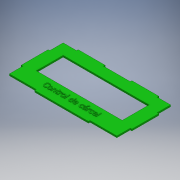
# Autodesk Inventor part: Control Frontal
Saved by Autodesk Inventor 2018 (Build 220112000, 112)
## iProperties
Created: 2020-03-09
Part Number: Control Frontal
Material: Genérico
Document SubType Name: Modeling
Designer: joser
Density: 1 g/cm^3
Appearance: Verde oscuro
Author: joser
Autodesk Inventor part; units mm, degrees
ref_plane "YZ Plane" through (0, 0, 0) normal (1, 0, 0) x (0, 1, 0)
ref_plane "XZ Plane" through (0, 0, 0) normal (0, 1, 0) x (-1, 0, 0)
ref_plane "XY Plane" through (0, 0, 0) normal (0, 0, 1) x (1, 0, 0)
sketch "Boceto1" plane through (0, 0, 0) normal (0, 0, 1) x (1, 0, 0)
  line L0 (-150, -3) -> (-50, -3)
  line L1 (-150, -3) -> (-150, 0)
  line L2 (-50, 0) -> (-50, -3)
  line L3 (-200, 0) -> (-150, 0)
  line L4 (-50, 0) -> (0, 0)
  line L5 (-180, 80) -> (-20, 80)
  line L6 (-20, 80) -> (-20, 30)
  line L7 (-20, 30) -> (-180, 30)
  line L8 (-180, 30) -> (-180, 80)
  line L9 (-200, 75) -> (-203, 75)
  line L10 (-203, 75) -> (-203, 25)
  line L11 (-203, 25) -> (-200, 25)
  line L12 (-200, 100) -> (-200, 75)
  line L13 (-200, 25) -> (-200, 0)
  line L14 (0, 75) -> (3, 75)
  line L15 (3, 75) -> (3, 25)
  line L16 (3, 25) -> (0, 25)
  line L17 (0, 75) -> (0, 100)
  line L18 (0, 0) -> (0, 25)
  line L19 (-175, 100) -> (-175, 103)
  line L20 (-175, 103) -> (-125, 103)
  line L21 (-125, 103) -> (-125, 100)
  line L22 (-75, 100) -> (-75, 103)
  line L23 (-75, 103) -> (-25, 103)
  line L24 (-25, 103) -> (-25, 100)
  line L25 (-175, 100) -> (-200, 100)
  line L26 (0, 100) -> (-25, 100)
  line L27 (-75, 100) -> (-125, 100)
  dimension "d11" = 160
  dimension "d12" = 50
  dimension "d15" = 3
  dimension "d16" = 50
  dimension "d19" = 20
  dimension "d20" = 50
  dimension "d21" = 50
  dimension "d22" = 3
  dimension "d23" = 200
  dimension "d24" = 50
  dimension "d25" = 3
  dimension "d26" = 50
  dimension "d27" = 50
  dimension "d28" = 50
  dimension "d35" = 20
  dimension "d41" = 25
  dimension "d42" = 3
  dimension "d43" = 25
  dimension "d45" = 100
  constraints: 56 end point, 16 perpendicular, 8 parallel, 6 collinear, 6 horizontal, 2 point on line, 2 vertical, 1 coincident
  measures "d11" distance between parallel lines of L6 L8
  measures "d12" distance between parallel lines of L7 L5
  measures "d15" distance between parallel lines of L12 L10
  measures "d16" distance between parallel lines of L11 L9
  measures "d19" distance between parallel lines of L12 L8
  measures "d20" distance between parallel lines of L1 L13
  measures "d21" distance between parallel lines of L16 L14
  measures "d22" distance between parallel lines of L17 L15
  measures "d23" distance between parallel lines of L17 L12
  measures "d24" distance between parallel lines of L18 L2
  measures "d25" distance between parallel lines of L25 L20
  measures "d26" distance between parallel lines of L21 L19
  measures "d27" distance between parallel lines of L24 L22
  measures "d28" distance between parallel lines of L21 L22
  measures "d35" distance between parallel lines of L25 L5
  measures "d41" distance between parallel lines of L17 L24
  measures "d42" distance between parallel lines of L3 L0
  measures "d43" distance between parallel lines of L3 L11
  measures "d45" distance between parallel lines of L4 L26
extrude "Extrusión1" add sketch "Boceto1" along normal blind 3
sketch "Boceto2" plane through (0, 0, 3) normal (0, 0, 1) x (1, 0, 0)
  line L0 (-175, 26.15) -> (-25, 26.15) construction
  line L1 (-25, 26.15) -> (-25, 7) construction
  line L2 (-25, 7) -> (-175, 7) construction
  line L3 (-175, 7) -> (-175, 26.15) construction
  line L4 (0, 0) -> (0, 25) projected
  line L5 (-150, -3) -> (-50, -3) projected
  spline S0 degree 2 poles (-146.1993, 10.874) (-147.1718, 10.874) (-148.8169, 11.5304) (-149.4165, 12.1868) knots 0 0 0 1 2 2 2
  spline S1 degree 2 poles (-149.4165, 12.1868) (-150.0162, 12.8351) (-150.6726, 14.78) (-150.6726, 16.0442) knots 0 0 0 1 2 2 2
  spline S2 degree 2 poles (-150.6726, 16.0442) (-150.6726, 17.3003) (-150.0324, 19.1641) (-149.4246, 19.853) knots 0 0 0 1 2 2 2
  spline S3 degree 2 poles (-149.4246, 19.853) (-148.825, 20.5256) (-147.188, 21.2306) (-146.175, 21.2306) knots 0 0 0 1 2 2 2
  spline S4 degree 2 poles (-146.175, 21.2306) (-145.6726, 21.2306) (-144.7893, 21.0847) (-144.4165, 20.9713) knots 0 0 0 1 2 2 2
  spline S5 degree 2 poles (-144.4165, 20.9713) (-144.0924, 20.8659) (-143.4198, 20.5661) (-143.0875, 20.3878) knots 0 0 0 1 2 2 2
  line L6 (-143.0875, 20.3878) -> (-143.0875, 18.7833)
  line L7 (-143.0875, 18.7833) -> (-143.1929, 18.7833)
  spline S6 degree 2 poles (-143.1929, 18.7833) (-143.3711, 18.9453) (-143.9222, 19.3992) (-144.3193, 19.618) knots 0 0 0 1 2 2 2
  spline S7 degree 2 poles (-144.3193, 19.618) (-144.7002, 19.8287) (-145.5997, 20.0961) (-146.1831, 20.0961) knots 0 0 0 1 2 2 2
  spline S8 degree 2 poles (-146.1831, 20.0961) (-146.8233, 20.0961) (-147.966, 19.5693) (-148.3955, 19.0669) knots 0 0 0 1 2 2 2
  spline S9 degree 2 poles (-148.3955, 19.0669) (-148.8169, 18.5564) (-149.2869, 17.0086) (-149.2869, 16.0442) knots 0 0 0 1 2 2 2
  spline S10 degree 2 poles (-149.2869, 16.0442) (-149.2869, 15.015) (-148.7925, 13.5321) (-148.363, 13.0215) knots 0 0 0 1 2 2 2
  spline S11 degree 2 poles (-148.363, 13.0215) (-147.9417, 12.5272) (-146.8152, 12.0248) (-146.1831, 12.0248) knots 0 0 0 1 2 2 2
  spline S12 degree 2 poles (-146.1831, 12.0248) (-145.6078, 12.0248) (-144.6272, 12.3084) (-144.2464, 12.5191) knots 0 0 0 1 2 2 2
  spline S13 degree 2 poles (-144.2464, 12.5191) (-143.8817, 12.7298) (-143.3387, 13.1674) (-143.1848, 13.3214) knots 0 0 0 1 2 2 2
  line L8 (-143.1848, 13.3214) -> (-143.0875, 13.3214)
  line L9 (-143.0875, 13.3214) -> (-143.0875, 11.733)
  spline S14 degree 2 poles (-143.0875, 11.733) (-143.4198, 11.5791) (-144.0032, 11.2954) (-144.4165, 11.1658) knots 0 0 0 1 2 2 2
  spline S15 degree 2 poles (-144.4165, 11.1658) (-144.8541, 11.0199) (-145.5997, 10.874) (-146.1993, 10.874) knots 0 0 0 1 2 2 2
  spline S16 degree 2 poles (-135.778, 14.8043) (-135.778, 12.9081) (-137.6013, 10.8416) (-139.1248, 10.8416) knots 0 0 0 1 2 2 2
  spline S17 degree 2 poles (-139.1248, 10.8416) (-140.6888, 10.8416) (-142.4797, 12.9729) (-142.4797, 14.8043) knots 0 0 0 1 2 2 2
  spline S18 degree 2 poles (-142.4797, 14.8043) (-142.4797, 16.6844) (-140.6321, 18.7671) (-139.1248, 18.7671) knots 0 0 0 1 2 2 2
  spline S19 degree 2 poles (-139.1248, 18.7671) (-137.6013, 18.7671) (-135.778, 16.6925) (-135.778, 14.8043) knots 0 0 0 1 2 2 2
  spline S20 degree 2 poles (-137.0827, 14.8043) (-137.0827, 16.263) (-138.1442, 17.6812) (-139.1248, 17.6812) knots 0 0 0 1 2 2 2
  spline S21 degree 2 poles (-139.1248, 17.6812) (-140.1053, 17.6812) (-141.175, 16.263) (-141.175, 14.8043) knots 0 0 0 1 2 2 2
  spline S22 degree 2 poles (-141.175, 14.8043) (-141.175, 13.3862) (-140.1053, 11.9275) (-139.1248, 11.9275) knots 0 0 0 1 2 2 2
  spline S23 degree 2 poles (-139.1248, 11.9275) (-138.1523, 11.9275) (-137.0827, 13.3619) (-137.0827, 14.8043) knots 0 0 0 1 2 2 2
  line L10 (-128.5899, 11.0523) -> (-129.8541, 11.0523)
  line L11 (-129.8541, 11.0523) -> (-129.8541, 15.3311)
  spline S24 degree 2 poles (-129.8541, 15.3311) (-129.8541, 15.8497) (-129.9514, 16.7411) (-130.0972, 17.0086) knots 0 0 0 1 2 2 2
  spline S25 degree 2 poles (-130.0972, 17.0086) (-130.2512, 17.2922) (-130.8023, 17.5677) (-131.2723, 17.5677) knots 0 0 0 1 2 2 2
  spline S26 degree 2 poles (-131.2723, 17.5677) (-131.7423, 17.5677) (-132.7391, 17.0653) (-133.2172, 16.6601) knots 0 0 0 1 2 2 2
  line L12 (-133.2172, 16.6601) -> (-133.2172, 11.0523)
  line L13 (-133.2172, 11.0523) -> (-134.4814, 11.0523)
  line L14 (-134.4814, 11.0523) -> (-134.4814, 18.5564)
  line L15 (-134.4814, 18.5564) -> (-133.2172, 18.5564)
  line L16 (-133.2172, 18.5564) -> (-133.2172, 17.7217)
  spline S27 degree 2 poles (-133.2172, 17.7217) (-132.6499, 18.2322) (-131.5559, 18.7671) (-130.94, 18.7671) knots 0 0 0 1 2 2 2
  spline S28 degree 2 poles (-130.94, 18.7671) (-129.8379, 18.7671) (-128.5899, 17.3084) (-128.5899, 15.9227) knots 0 0 0 1 2 2 2
  line L17 (-128.5899, 15.9227) -> (-128.5899, 11.0523)
  spline S29 degree 2 poles (-124.5462, 10.9064) (-125.5754, 10.9064) (-126.7342, 12.0815) (-126.7342, 13.3538) knots 0 0 0 1 2 2 2
  line L18 (-126.7342, 13.3538) -> (-126.7342, 17.511)
  line L19 (-126.7342, 17.511) -> (-127.5851, 17.511)
  line L20 (-127.5851, 17.511) -> (-127.5851, 18.5564)
  line L21 (-127.5851, 18.5564) -> (-126.7342, 18.5564)
  line L22 (-126.7342, 18.5564) -> (-126.7342, 20.712)
  line L23 (-126.7342, 20.712) -> (-125.47, 20.712)
  line L24 (-125.47, 20.712) -> (-125.47, 18.5564)
  line L25 (-125.47, 18.5564) -> (-123.1442, 18.5564)
  line L26 (-123.1442, 18.5564) -> (-123.1442, 17.511)
  line L27 (-123.1442, 17.511) -> (-125.47, 17.511)
  line L28 (-125.47, 17.511) -> (-125.47, 13.9372)
  spline S30 degree 2 poles (-125.47, 13.9372) (-125.47, 13.37) (-125.4295, 12.746) (-125.2917, 12.4786) knots 0 0 0 1 2 2 2
  spline S31 degree 2 poles (-125.2917, 12.4786) (-125.1783, 12.2436) (-124.6677, 12.0086) (-124.2301, 12.0086) knots 0 0 0 1 2 2 2
  spline S32 degree 2 poles (-124.2301, 12.0086) (-123.9222, 12.0086) (-123.3468, 12.1949) (-123.2172, 12.2517) knots 0 0 0 1 2 2 2
  line L29 (-123.2172, 12.2517) -> (-123.1442, 12.2517)
  line L30 (-123.1442, 12.2517) -> (-123.1442, 11.1171)
  spline S33 degree 2 poles (-123.1442, 11.1171) (-123.5008, 11.0199) (-124.2301, 10.9064) (-124.5462, 10.9064) knots 0 0 0 1 2 2 2
  line L31 (-118.2334, 17.203) -> (-118.2982, 17.203)
  spline S34 degree 2 poles (-118.2982, 17.203) (-118.4441, 17.2436) (-118.7601, 17.2598) (-118.9789, 17.2598) knots 0 0 0 1 2 2 2
  spline S35 degree 2 poles (-118.9789, 17.2598) (-119.4895, 17.2598) (-120.4943, 16.8141) (-120.9481, 16.3765) knots 0 0 0 1 2 2 2
  line L32 (-120.9481, 16.3765) -> (-120.9481, 11.0523)
  line L33 (-120.9481, 11.0523) -> (-122.2123, 11.0523)
  line L34 (-122.2123, 11.0523) -> (-122.2123, 18.5564)
  line L35 (-122.2123, 18.5564) -> (-120.9481, 18.5564)
  line L36 (-120.9481, 18.5564) -> (-120.9481, 17.4381)
  spline S36 degree 2 poles (-120.9481, 17.4381) (-120.2593, 18.0539) (-119.2301, 18.5564) (-118.7439, 18.5564) knots 0 0 0 1 2 2 2
  spline S37 degree 2 poles (-118.7439, 18.5564) (-118.5494, 18.5564) (-118.3549, 18.5402) (-118.2334, 18.5158) knots 0 0 0 1 2 2 2
  line L37 (-118.2334, 18.5158) -> (-118.2334, 17.203)
  spline S38 degree 2 poles (-111.0859, 14.8043) (-111.0859, 12.9081) (-112.9092, 10.8416) (-114.4327, 10.8416) knots 0 0 0 1 2 2 2
  spline S39 degree 2 poles (-114.4327, 10.8416) (-115.9968, 10.8416) (-117.7877, 12.9729) (-117.7877, 14.8043) knots 0 0 0 1 2 2 2
  spline S40 degree 2 poles (-117.7877, 14.8043) (-117.7877, 16.6844) (-115.94, 18.7671) (-114.4327, 18.7671) knots 0 0 0 1 2 2 2
  spline S41 degree 2 poles (-114.4327, 18.7671) (-112.9092, 18.7671) (-111.0859, 16.6925) (-111.0859, 14.8043) knots 0 0 0 1 2 2 2
  spline S42 degree 2 poles (-112.3906, 14.8043) (-112.3906, 16.263) (-113.4522, 17.6812) (-114.4327, 17.6812) knots 0 0 0 1 2 2 2
  spline S43 degree 2 poles (-114.4327, 17.6812) (-115.4133, 17.6812) (-116.483, 16.263) (-116.483, 14.8043) knots 0 0 0 1 2 2 2
  spline S44 degree 2 poles (-116.483, 14.8043) (-116.483, 13.3862) (-115.4133, 11.9275) (-114.4327, 11.9275) knots 0 0 0 1 2 2 2
  spline S45 degree 2 poles (-114.4327, 11.9275) (-113.4603, 11.9275) (-112.3906, 13.3619) (-112.3906, 14.8043) knots 0 0 0 1 2 2 2
  line L38 (-108.5008, 11.0523) -> (-109.765, 11.0523)
  line L39 (-109.765, 11.0523) -> (-109.765, 21.498)
  line L40 (-109.765, 21.498) -> (-108.5008, 21.498)
  line L41 (-108.5008, 21.498) -> (-108.5008, 11.0523)
  line L42 (-96.5802, 11.0523) -> (-97.8444, 11.0523)
  line L43 (-97.8444, 11.0523) -> (-97.8444, 11.8141)
  spline S46 degree 2 poles (-97.8444, 11.8141) (-98.1361, 11.571) (-98.5656, 11.2468) (-98.8574, 11.109) knots 0 0 0 1 2 2 2
  spline S47 degree 2 poles (-98.8574, 11.109) (-99.1248, 10.9794) (-99.7002, 10.8416) (-100.081, 10.8416) knots 0 0 0 1 2 2 2
  spline S48 degree 2 poles (-100.081, 10.8416) (-100.6969, 10.8416) (-101.7342, 11.3522) (-102.0989, 11.8465) knots 0 0 0 1 2 2 2
  spline S49 degree 2 poles (-102.0989, 11.8465) (-102.4635, 12.3408) (-102.8687, 13.7995) (-102.8687, 14.7476) knots 0 0 0 1 2 2 2
  spline S50 degree 2 poles (-102.8687, 14.7476) (-102.8687, 15.7363) (-102.3582, 17.1787) (-101.9125, 17.7217) knots 0 0 0 1 2 2 2
  spline S51 degree 2 poles (-101.9125, 17.7217) (-101.4992, 18.2079) (-100.3404, 18.7671) (-99.7002, 18.7671) knots 0 0 0 1 2 2 2
  spline S52 degree 2 poles (-99.7002, 18.7671) (-99.141, 18.7671) (-98.3063, 18.5158) (-97.8444, 18.2565) knots 0 0 0 1 2 2 2
  line L44 (-97.8444, 18.2565) -> (-97.8444, 21.498)
  line L45 (-97.8444, 21.498) -> (-96.5802, 21.498)
  line L46 (-96.5802, 21.498) -> (-96.5802, 11.0523)
  line L47 (-97.8444, 12.8757) -> (-97.8444, 17.2111)
  spline S53 degree 2 poles (-97.8444, 17.2111) (-98.3144, 17.4381) (-99.06, 17.6082) (-99.4895, 17.6082) knots 0 0 0 1 2 2 2
  spline S54 degree 2 poles (-99.4895, 17.6082) (-100.4619, 17.6082) (-101.564, 16.1496) (-101.564, 14.7719) knots 0 0 0 1 2 2 2
  spline S55 degree 2 poles (-101.564, 14.7719) (-101.564, 13.4429) (-100.7212, 12.041) (-99.7893, 12.041) knots 0 0 0 1 2 2 2
  spline S56 degree 2 poles (-99.7893, 12.041) (-99.295, 12.041) (-98.2901, 12.4948) (-97.8444, 12.8757) knots 0 0 0 1 2 2 2
  spline S57 degree 2 poles (-91.4911, 10.8821) (-93.2901, 10.8821) (-95.2674, 12.9) (-95.2674, 14.7638) knots 0 0 0 1 2 2 2
  spline S58 degree 2 poles (-95.2674, 14.7638) (-95.2674, 16.5953) (-93.3468, 18.7671) (-91.799, 18.7671) knots 0 0 0 1 2 2 2
  spline S59 degree 2 poles (-91.799, 18.7671) (-91.1021, 18.7671) (-90.0243, 18.3619) (-89.6272, 17.9324) knots 0 0 0 1 2 2 2
  spline S60 degree 2 poles (-89.6272, 17.9324) (-89.222, 17.5029) (-88.7925, 16.263) (-88.7925, 15.3635) knots 0 0 0 1 2 2 2
  line L48 (-88.7925, 15.3635) -> (-88.7925, 14.6747)
  line L49 (-88.7925, 14.6747) -> (-93.987, 14.6747)
  spline S61 degree 2 poles (-93.987, 14.6747) (-93.987, 13.37) (-92.6742, 11.9842) (-91.5073, 11.9842) knots 0 0 0 1 2 2 2
  spline S62 degree 2 poles (-91.5073, 11.9842) (-91.094, 11.9842) (-90.2917, 12.1706) (-89.9676, 12.3165) knots 0 0 0 1 2 2 2
  spline S63 degree 2 poles (-89.9676, 12.3165) (-89.6272, 12.4786) (-89.1572, 12.7622) (-89.0032, 12.8919) knots 0 0 0 1 2 2 2
  line L50 (-89.0032, 12.8919) -> (-88.9303, 12.8919)
  line L51 (-88.9303, 12.8919) -> (-88.9303, 11.5142)
  spline S64 degree 2 poles (-88.9303, 11.5142) (-89.1491, 11.4251) (-89.8136, 11.1658) (-90.0729, 11.0928) knots 0 0 0 1 2 2 2
  spline S65 degree 2 poles (-90.0729, 11.0928) (-90.4376, 10.9875) (-91.0373, 10.8821) (-91.4911, 10.8821) knots 0 0 0 1 2 2 2
  spline S66 degree 2 poles (-90.0243, 15.639) (-90.0405, 16.1496) (-90.2512, 16.8951) (-90.4538, 17.1463) knots 0 0 0 1 2 2 2
  spline S67 degree 2 poles (-90.4538, 17.1463) (-90.6726, 17.4299) (-91.3614, 17.7298) (-91.872, 17.7298) knots 0 0 0 1 2 2 2
  spline S68 degree 2 poles (-91.872, 17.7298) (-92.3744, 17.7298) (-93.0794, 17.4299) (-93.3711, 17.1382) knots 0 0 0 1 2 2 2
  spline S69 degree 2 poles (-93.3711, 17.1382) (-93.6548, 16.8384) (-93.9465, 16.1171) (-93.987, 15.639) knots 0 0 0 1 2 2 2
  line L52 (-93.987, 15.639) -> (-90.0243, 15.639)
  spline S70 degree 2 poles (-80.235, 10.8821) (-81.013, 10.8821) (-82.3015, 11.3603) (-82.7634, 11.8465) knots 0 0 0 1 2 2 2
  spline S71 degree 2 poles (-82.7634, 11.8465) (-83.2253, 12.3246) (-83.7358, 13.7995) (-83.7358, 14.7881) knots 0 0 0 1 2 2 2
  spline S72 degree 2 poles (-83.7358, 14.7881) (-83.7358, 15.7768) (-83.2091, 17.2193) (-82.7634, 17.7055) knots 0 0 0 1 2 2 2
  spline S73 degree 2 poles (-82.7634, 17.7055) (-82.3177, 18.1998) (-80.9968, 18.7265) (-80.235, 18.7265) knots 0 0 0 1 2 2 2
  spline S74 degree 2 poles (-80.235, 18.7265) (-79.6191, 18.7265) (-78.4684, 18.3781) (-78.0227, 18.1512) knots 0 0 0 1 2 2 2
  line L53 (-78.0227, 18.1512) -> (-78.0227, 16.733)
  line L54 (-78.0227, 16.733) -> (-78.0956, 16.733)
  spline S75 degree 2 poles (-78.0956, 16.733) (-78.2334, 16.8465) (-78.6548, 17.1382) (-78.9546, 17.2922) knots 0 0 0 1 2 2 2
  spline S76 degree 2 poles (-78.9546, 17.2922) (-79.222, 17.4218) (-79.9352, 17.6244) (-80.2593, 17.6244) knots 0 0 0 1 2 2 2
  spline S77 degree 2 poles (-80.2593, 17.6244) (-81.2399, 17.6244) (-82.4311, 16.1415) (-82.4311, 14.7881) knots 0 0 0 1 2 2 2
  spline S78 degree 2 poles (-82.4311, 14.7881) (-82.4311, 13.4672) (-81.2804, 11.9842) (-80.2593, 11.9842) knots 0 0 0 1 2 2 2
  spline S79 degree 2 poles (-80.2593, 11.9842) (-79.6434, 11.9842) (-78.5251, 12.4948) (-78.0956, 12.8919) knots 0 0 0 1 2 2 2
  line L55 (-78.0956, 12.8919) -> (-78.0227, 12.8919)
  line L56 (-78.0227, 12.8919) -> (-78.0227, 11.4737)
  spline S80 degree 2 poles (-78.0227, 11.4737) (-78.2091, 11.3846) (-78.7763, 11.1334) (-79.0032, 11.0766) knots 0 0 0 1 2 2 2
  spline S81 degree 2 poles (-79.0032, 11.0766) (-79.3274, 10.9794) (-79.8379, 10.8821) (-80.235, 10.8821) knots 0 0 0 1 2 2 2
  spline S82 degree 2 poles (-72.6904, 11.8465) (-72.8444, 11.733) (-73.363, 11.3278) (-73.6062, 11.2063) knots 0 0 0 1 2 2 2
  spline S83 degree 2 poles (-73.6062, 11.2063) (-73.9384, 11.028) (-74.5624, 10.8416) (-75.1297, 10.8416) knots 0 0 0 1 2 2 2
  spline S84 degree 2 poles (-75.1297, 10.8416) (-75.5916, 10.8416) (-76.4263, 11.1901) (-76.7423, 11.5061) knots 0 0 0 1 2 2 2
  spline S85 degree 2 poles (-76.7423, 11.5061) (-77.0421, 11.8141) (-77.4068, 12.7217) (-77.4068, 13.2241) knots 0 0 0 1 2 2 2
  spline S86 degree 2 poles (-77.4068, 13.2241) (-77.4068, 14.0021) (-76.7504, 15.1042) (-76.0373, 15.4202) knots 0 0 0 1 2 2 2
  spline S87 degree 2 poles (-76.0373, 15.4202) (-75.4052, 15.712) (-73.6872, 15.9308) (-72.6904, 15.9875) knots 0 0 0 1 2 2 2
  line L57 (-72.6904, 15.9875) -> (-72.6904, 16.2306)
  spline S88 degree 2 poles (-72.6904, 16.2306) (-72.6904, 16.6682) (-72.9579, 17.2111) (-73.201, 17.3651) knots 0 0 0 1 2 2 2
  spline S89 degree 2 poles (-73.201, 17.3651) (-73.4441, 17.5191) (-74.141, 17.6163) (-74.5138, 17.6163) knots 0 0 0 1 2 2 2
  spline S90 degree 2 poles (-74.5138, 17.6163) (-74.9514, 17.6163) (-76.1345, 17.357) (-76.7261, 17.1058) knots 0 0 0 1 2 2 2
  line L58 (-76.7261, 17.1058) -> (-76.799, 17.1058)
  line L59 (-76.799, 17.1058) -> (-76.799, 18.3943)
  spline S91 degree 2 poles (-76.799, 18.3943) (-76.4506, 18.4915) (-75.1459, 18.7346) (-74.5057, 18.7346) knots 0 0 0 1 2 2 2
  spline S92 degree 2 poles (-74.5057, 18.7346) (-73.7277, 18.7346) (-72.6661, 18.4915) (-72.2447, 18.1755) knots 0 0 0 1 2 2 2
  spline S93 degree 2 poles (-72.2447, 18.1755) (-71.8314, 17.8675) (-71.4263, 16.887) (-71.4263, 16.182) knots 0 0 0 1 2 2 2
  line L60 (-71.4263, 16.182) -> (-71.4263, 11.0523)
  line L61 (-71.4263, 11.0523) -> (-72.6904, 11.0523)
  line L62 (-72.6904, 11.0523) -> (-72.6904, 11.8465)
  line L63 (-72.6904, 12.9) -> (-72.6904, 14.9826)
  spline S94 degree 2 poles (-72.6904, 14.9826) (-73.1442, 14.9421) (-74.5138, 14.8043) (-74.9433, 14.6747) knots 0 0 0 1 2 2 2
  spline S95 degree 2 poles (-74.9433, 14.6747) (-75.4457, 14.5207) (-76.1021, 13.8805) (-76.1021, 13.3133) knots 0 0 0 1 2 2 2
  spline S96 degree 2 poles (-76.1021, 13.3133) (-76.1021, 12.665) (-75.3728, 12.0086) (-74.6758, 12.0086) knots 0 0 0 1 2 2 2
  spline S97 degree 2 poles (-74.6758, 12.0086) (-74.0843, 12.0086) (-73.1118, 12.5191) (-72.6904, 12.9) knots 0 0 0 1 2 2 2
  line L64 (-72.1718, 22.3084) -> (-74.0032, 19.7962)
  line L65 (-74.0032, 19.7962) -> (-75.0081, 19.7962)
  line L66 (-75.0081, 19.7962) -> (-73.8087, 22.3084)
  line L67 (-73.8087, 22.3084) -> (-72.1718, 22.3084)
  line L68 (-65.6726, 17.203) -> (-65.7374, 17.203)
  spline S98 degree 2 poles (-65.7374, 17.203) (-65.8833, 17.2436) (-66.1993, 17.2598) (-66.4181, 17.2598) knots 0 0 0 1 2 2 2
  spline S99 degree 2 poles (-66.4181, 17.2598) (-66.9287, 17.2598) (-67.9335, 16.8141) (-68.3874, 16.3765) knots 0 0 0 1 2 2 2
  line L69 (-68.3874, 16.3765) -> (-68.3874, 11.0523)
  line L70 (-68.3874, 11.0523) -> (-69.6515, 11.0523)
  line L71 (-69.6515, 11.0523) -> (-69.6515, 18.5564)
  line L72 (-69.6515, 18.5564) -> (-68.3874, 18.5564)
  line L73 (-68.3874, 18.5564) -> (-68.3874, 17.4381)
  spline S100 degree 2 poles (-68.3874, 17.4381) (-67.6985, 18.0539) (-66.6694, 18.5564) (-66.1831, 18.5564) knots 0 0 0 1 2 2 2
  spline S101 degree 2 poles (-66.1831, 18.5564) (-65.9887, 18.5564) (-65.7942, 18.5402) (-65.6726, 18.5158) knots 0 0 0 1 2 2 2
  line L74 (-65.6726, 18.5158) -> (-65.6726, 17.203)
  spline S102 degree 2 poles (-61.7099, 10.8821) (-62.4878, 10.8821) (-63.7763, 11.3603) (-64.2382, 11.8465) knots 0 0 0 1 2 2 2
  spline S103 degree 2 poles (-64.2382, 11.8465) (-64.7002, 12.3246) (-65.2107, 13.7995) (-65.2107, 14.7881) knots 0 0 0 1 2 2 2
  spline S104 degree 2 poles (-65.2107, 14.7881) (-65.2107, 15.7768) (-64.684, 17.2193) (-64.2382, 17.7055) knots 0 0 0 1 2 2 2
  spline S105 degree 2 poles (-64.2382, 17.7055) (-63.7925, 18.1998) (-62.4716, 18.7265) (-61.7099, 18.7265) knots 0 0 0 1 2 2 2
  spline S106 degree 2 poles (-61.7099, 18.7265) (-61.094, 18.7265) (-59.9433, 18.3781) (-59.4976, 18.1512) knots 0 0 0 1 2 2 2
  line L75 (-59.4976, 18.1512) -> (-59.4976, 16.733)
  line L76 (-59.4976, 16.733) -> (-59.5705, 16.733)
  spline S107 degree 2 poles (-59.5705, 16.733) (-59.7083, 16.8465) (-60.1297, 17.1382) (-60.4295, 17.2922) knots 0 0 0 1 2 2 2
  spline S108 degree 2 poles (-60.4295, 17.2922) (-60.6969, 17.4218) (-61.41, 17.6244) (-61.7342, 17.6244) knots 0 0 0 1 2 2 2
  spline S109 degree 2 poles (-61.7342, 17.6244) (-62.7147, 17.6244) (-63.906, 16.1415) (-63.906, 14.7881) knots 0 0 0 1 2 2 2
  spline S110 degree 2 poles (-63.906, 14.7881) (-63.906, 13.4672) (-62.7553, 11.9842) (-61.7342, 11.9842) knots 0 0 0 1 2 2 2
  spline S111 degree 2 poles (-61.7342, 11.9842) (-61.1183, 11.9842) (-60, 12.4948) (-59.5705, 12.8919) knots 0 0 0 1 2 2 2
  line L77 (-59.5705, 12.8919) -> (-59.4976, 12.8919)
  line L78 (-59.4976, 12.8919) -> (-59.4976, 11.4737)
  spline S112 degree 2 poles (-59.4976, 11.4737) (-59.684, 11.3846) (-60.2512, 11.1334) (-60.4781, 11.0766) knots 0 0 0 1 2 2 2
  spline S113 degree 2 poles (-60.4781, 11.0766) (-60.8023, 10.9794) (-61.3128, 10.8821) (-61.7099, 10.8821) knots 0 0 0 1 2 2 2
  spline S114 degree 2 poles (-55.0891, 10.8821) (-56.8882, 10.8821) (-58.8655, 12.9) (-58.8655, 14.7638) knots 0 0 0 1 2 2 2
  spline S115 degree 2 poles (-58.8655, 14.7638) (-58.8655, 16.5953) (-56.9449, 18.7671) (-55.3971, 18.7671) knots 0 0 0 1 2 2 2
  spline S116 degree 2 poles (-55.3971, 18.7671) (-54.7002, 18.7671) (-53.6224, 18.3619) (-53.2253, 17.9324) knots 0 0 0 1 2 2 2
  spline S117 degree 2 poles (-53.2253, 17.9324) (-52.8201, 17.5029) (-52.3906, 16.263) (-52.3906, 15.3635) knots 0 0 0 1 2 2 2
  line L79 (-52.3906, 15.3635) -> (-52.3906, 14.6747)
  line L80 (-52.3906, 14.6747) -> (-57.5851, 14.6747)
  spline S118 degree 2 poles (-57.5851, 14.6747) (-57.5851, 13.37) (-56.2723, 11.9842) (-55.1053, 11.9842) knots 0 0 0 1 2 2 2
  spline S119 degree 2 poles (-55.1053, 11.9842) (-54.6921, 11.9842) (-53.8898, 12.1706) (-53.5656, 12.3165) knots 0 0 0 1 2 2 2
  spline S120 degree 2 poles (-53.5656, 12.3165) (-53.2253, 12.4786) (-52.7553, 12.7622) (-52.6013, 12.8919) knots 0 0 0 1 2 2 2
  line L81 (-52.6013, 12.8919) -> (-52.5284, 12.8919)
  line L82 (-52.5284, 12.8919) -> (-52.5284, 11.5142)
  spline S121 degree 2 poles (-52.5284, 11.5142) (-52.7472, 11.4251) (-53.4117, 11.1658) (-53.671, 11.0928) knots 0 0 0 1 2 2 2
  spline S122 degree 2 poles (-53.671, 11.0928) (-54.0357, 10.9875) (-54.6353, 10.8821) (-55.0891, 10.8821) knots 0 0 0 1 2 2 2
  spline S123 degree 2 poles (-53.6224, 15.639) (-53.6386, 16.1496) (-53.8493, 16.8951) (-54.0519, 17.1463) knots 0 0 0 1 2 2 2
  spline S124 degree 2 poles (-54.0519, 17.1463) (-54.2707, 17.4299) (-54.9595, 17.7298) (-55.47, 17.7298) knots 0 0 0 1 2 2 2
  spline S125 degree 2 poles (-55.47, 17.7298) (-55.9724, 17.7298) (-56.6775, 17.4299) (-56.9692, 17.1382) knots 0 0 0 1 2 2 2
  spline S126 degree 2 poles (-56.9692, 17.1382) (-57.2528, 16.8384) (-57.5446, 16.1171) (-57.5851, 15.639) knots 0 0 0 1 2 2 2
  line L83 (-57.5851, 15.639) -> (-53.6224, 15.639)
  line L84 (-49.8217, 11.0523) -> (-51.0859, 11.0523)
  line L85 (-51.0859, 11.0523) -> (-51.0859, 21.498)
  line L86 (-51.0859, 21.498) -> (-49.8217, 21.498)
  line L87 (-49.8217, 21.498) -> (-49.8217, 11.0523)
  dimension "d36" = 150
  dimension "d37" = 25
  dimension "d38" = 10
  constraints: 2 other
  measures "d36" distance between parallel lines of L3 L1
  measures "d37" distance between parallel lines of L4 L1
  measures "d38" distance between parallel lines of L5 L2
extrude "Extrusión2" add sketch "Boceto2" along normal blind 1
